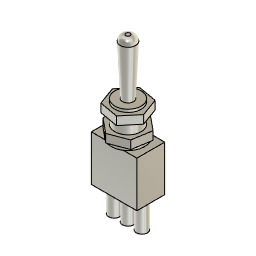
Zusammenbau V2 v20 (Autodesk Fusion 360 archive; units mm, degrees)
design "Schalter"
Autodesk Fusion 360 part; units mm, degrees
sketch "Skizze1" plane through (0, 0, 0) normal (0, 0, 1) x (1, 0, 0)
  line L0 (0, 0) -> (8.2, 0)
  line L1 (8.2, 0) -> (8.2, 5)
  line L2 (8.2, 5) -> (0, 5)
  line L3 (0, 5) -> (0, 0)
  dimension "d1" = 8.2
  dimension "d2" = 5
  constraint horizontal L0
  constraint vertical L1
  constraint horizontal L2
  constraint vertical L3
  constraint coincident L0.start L3.end
  measures "d1" distance of L0.start L0.end
  measures "d2" distance of L0.start L2.end
extrude "Extrusion1" add sketch "Skizze1" along normal blind 8.2
sketch "Skizze2" plane through (0, 0, 8.2) normal (0, 0, 1) x (-1, 0, 0)
  line L0 (0, -5) -> (0, 0)
  line L1 (0, 0) -> (-8.2, 0)
  line L2 (-8.2, 0) -> (-8.2, -5)
  line L3 (-8.2, -5) -> (0, -5)
  circle A0 centre (-4.1, -2.5) radius 3
  dimension "d5" = 6
  dimension "d6" = 2.5
  dimension "d38" = 4.1
  measures "d5" diameter of A0
  measures "d6" distance of L1 A0.centre
  measures "d38" distance of L0 A0.centre
extrude "Extrusion2" add sketch "Skizze2" along normal blind 0.5 contours L3 A0 | L1 L3 A0 | L1 A0
sketch "Skizze3" plane through (0, 0, 8.7) normal (0, 0, 1) x (-1, 0, 0)
  circle A0 centre (-4.1, -2.5) radius 3
  circle A1 centre (-4.1, -2.5) radius 2.375
  dimension "d9" = 4.75
  constraint concentric A0 A1
  measures "d9" diameter of A1
extrude "Extrusion3" add sketch "Skizze3" along normal blind 5.5 contours A1
sketch "Skizze4" plane through (0, 0, 14.2) normal (0, 0, 1) x (-1, 0, 0)
  circle A0 centre (-4.1, -2.5) radius 2.375
  circle A1 centre (-4.1, -2.5) radius 1.25
  dimension "d12" = 2.5
  constraint concentric A0 A1
  measures "d12" diameter of A1
sketch "Skizze5" plane through (0, 0, 0) normal (0, 0, -1) x (1, 0, 0)
  line L0 (0, 0) -> (0, -5)
  line L1 (0, -5) -> (8.2, -5)
  line L2 (8.2, -5) -> (8.2, 0)
  line L3 (8.2, 0) -> (0, 0)
  circle A0 centre (4.1, -2.5) radius 1
  circle A1 centre (6.6, -2.5) radius 1
  circle A2 centre (1.6, -2.5) radius 1
  dimension "d17" = 2
  dimension "d18" = 2.5
  dimension "d21" = 2.5
  dimension "d22" = 0
  dimension "d25" = -2.5
  dimension "d26" = 0
  dimension "d39" = 4.1
  measures "d17" diameter of A0
  measures "d18" distance of L1 A0.centre
  measures "d39" distance of L0 A0.centre
extrude "Extrusion5" add sketch "Skizze5" along normal blind 5 contours A0 | A1 | A2
sketch "Skizze6" plane through (0, 0, 8.7) normal (0, 0, 1) x (-1, 0, 0)
  circle A0 centre (-4.1, -2.5) radius 2.375
  circle A1 centre (-4.1, -2.5) radius 3
  line L0 (-7.3757, -3.7328) -> (-4.6702, -5.9532)
  line L1 (-4.6702, -5.9532) -> (-1.3945, -4.7204)
  line L2 (-1.3945, -4.7204) -> (-0.8243, -1.2672)
  line L3 (-0.8243, -1.2672) -> (-3.5298, 0.9532)
  line L4 (-3.5298, 0.9532) -> (-6.8055, -0.2796)
  line L5 (-6.8055, -0.2796) -> (-7.3757, -3.7328)
  point P0 (-4.1, -2.5)
  dimension "d29" = 3.5
  constraint coincident P0 A0.centre
  measures "d29" distance of L0.start P0
extrude "Extrusion6" add sketch "Skizze6" along normal blind 1.5 contours A1 | L0 L1 L2 L3 L4 L5
ref_plane "Arbeitsebene1" through (4.1, 2.5, 12.2) normal (0, 0, 1) x (-1, 0, 0)
sketch "Skizze8" plane through (4.1, 2.5, 12.2) normal (0, 0, 1) x (1, 0, 0)
  line L0 (-1.1793, 3.2572) -> (-3.4105, 0.6073)
  line L1 (-3.4105, 0.6073) -> (-2.2311, -2.6499)
  line L2 (-2.2311, -2.6499) -> (1.1793, -3.2572)
  line L3 (1.1793, -3.2572) -> (3.4105, -0.6073)
  line L4 (3.4105, -0.6073) -> (2.2311, 2.6499)
  line L5 (2.2311, 2.6499) -> (-1.1793, 3.2572)
  dimension "d40" = 3
  measures "d40" distance of origin L5
extrude "Extrusion9" add sketch "Skizze8" along normal blind 1.5
sketch "Skizze9" plane through (0, 0, 14.2) normal (0, 0, 1) x (-1, 0, 0)
  circle A0 centre (-4.1, -2.5) radius 2.375
  circle A1 centre (-4.1, -2.5) radius 1
  dimension "d43" = 2
  constraint concentric A0 A1
  measures "d43" diameter of A1
extrude "Extrusion10" add sketch "Skizze9" along normal blind 10 draft 2.5 contours A1
fillet "Abrundung2" radius 1 1 edges at (5.4394, 1.9805, 24.2)

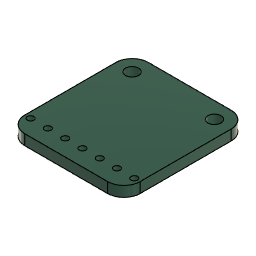
design "BME280"
Autodesk Fusion 360 part; units mm, degrees
sketch "Skizze1" plane through (0, 0, 0) normal (0, 0, 1) x (1, 0, 0)
  line L0 (2.5, 0) -> (15.28, 0)
  line L1 (17.78, 2.5) -> (17.78, 16.55)
  line L2 (15.28, 19.05) -> (2.5, 19.05)
  line L3 (0, 16.55) -> (0, 2.5)
  arc A0 (2.5, 19.05) -> (0, 16.55) centre (2.5, 16.55) ccw
  arc A1 (17.78, 16.55) -> (15.28, 19.05) centre (15.28, 16.55) ccw
  arc A2 (15.28, 0) -> (17.78, 2.5) centre (15.28, 2.5) ccw
  arc A3 (0, 2.5) -> (2.5, 0) centre (2.5, 2.5) ccw
  circle A4 centre (2.5, 16.55) radius 1
  circle A5 centre (15.2, 16.55) radius 1
  circle A6 centre (0.89, 2.5) radius 0.5
  circle A7 centre (3.5567, 2.5) radius 0.5
  circle A8 centre (6.2233, 2.5) radius 0.5
  circle A9 centre (8.89, 2.5) radius 0.5
  circle A10 centre (11.5567, 2.5) radius 0.5
  circle A11 centre (14.2233, 2.5) radius 0.5
  circle A12 centre (16.89, 2.5) radius 0.5
  point P0 (17.78, 0)
  dimension "d3" = 17.78
  dimension "d4" = 19.05
  dimension "d5" = 2.5
  dimension "d6" = 2
  dimension "d9" = 12.7
  dimension "d10" = 0
  dimension "d11" = 1
  dimension "d12" = 2.5
  dimension "d15" = 16
  dimension "d16" = 0
  dimension "d17" = 8.89
  constraint horizontal L0
  constraint vertical L1
  constraint horizontal L2
  constraint vertical L3
  constraint tangent L2 A0
  constraint tangent L3 A0
  constraint tangent L1 A1
  constraint tangent L2 A1
  constraint equal A0 A1
  constraint coincident P0 L0
  constraint coincident P0 L1
  constraint tangent L0 A2
  constraint tangent L1 A2
  constraint equal A0 A2
  constraint coincident origin L0
  constraint coincident origin L3
  constraint tangent L0 A3
  constraint tangent L3 A3
  constraint equal A0 A3
  constraint concentric A0 A4
  measures "d3" distance of origin P0
  measures "d4" distance of L0 L2
  measures "d5" radius of A0
  measures "d6" diameter of A4
  measures "d11" diameter of A6
  measures "d12" distance of L0 A6.centre
  measures "d17" distance of L3 A9.centre
extrude "Extrusion1" add sketch "Skizze1" along normal blind 1.6

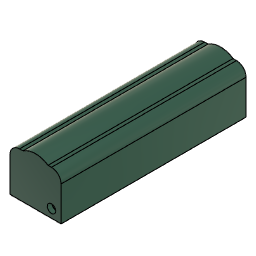
design "18650 Li-Ion Akku"
Autodesk Fusion 360 part; units mm, degrees
sketch "Skizze1" plane through (0, 0, 0) normal (0, 0, 1) x (1, 0, 0)
  line L0 (0, 0) -> (21.3, 0)
  line L1 (21.3, 0) -> (21.3, 77)
  line L2 (21.3, 77) -> (0, 77)
  line L3 (0, 77) -> (0, 0)
  dimension "d1" = 21.3
  dimension "d2" = 77
  constraint horizontal L0
  constraint vertical L1
  constraint horizontal L2
  constraint vertical L3
  constraint coincident L0.start L3.end
  measures "d1" distance of L0.start L0.end
  measures "d2" distance of L0.start L2.end
extrude "Extrusion1" add sketch "Skizze1" along normal blind 18.4
fillet "Abrundung1" radius 4 2 edges at (21.3, 38.5, 18.4) (0, 38.5, 18.4)
sketch "Skizze3" plane through (0, 0, 0) normal (0, -1, 0) x (1, 0, 0)
  arc A0 (4, 18.4) -> (0, 14.4) centre (4, 14.4) ccw
  line L0 (0, 14.4) -> (0, 0)
  line L1 (0, 0) -> (21.3, 0)
  line L2 (21.3, 0) -> (21.3, 14.4)
  arc A1 (21.3, 14.4) -> (17.3, 18.4) centre (17.3, 14.4) ccw
  line L3 (17.3, 18.4) -> (4, 18.4)
  circle A2 centre (10.65, 10.75) radius 9.25
  dimension "d10" = 18.5
  dimension "d11" = 10.75
  dimension "d12" = 10.65
  measures "d10" diameter of A2
  measures "d11" distance of L1 A2.centre
  measures "d12" distance of L0 A2.centre
extrude "Extrusion3" add sketch "Skizze3" against normal blind 77 contours L3 A2 picked at (9.7432, 18.797)
sketch "Skizze4" plane through (0, 0, 0) normal (0, -1, 0) x (1, 0, 0)
  arc A0 (4, 18.4) -> (0, 14.4) centre (4, 14.4) ccw
  line L0 (0, 14.4) -> (0, 0)
  line L1 (0, 0) -> (21.3, 0)
  line L2 (21.3, 0) -> (21.3, 14.4)
  arc A1 (21.3, 14.4) -> (17.3, 18.4) centre (17.3, 14.4) ccw
  line L3 (17.3, 18.4) -> (15.85, 18.4)
  arc A2 (15.85, 18.4) -> (5.45, 18.4) centre (10.65, 10.75) ccw
  line L4 (5.45, 18.4) -> (4, 18.4)
  circle A3 centre (17.3, 3.5) radius 1.75
  dimension "d15" = 3.5
  dimension "d16" = 4
  dimension "d17" = 3.5
  measures "d15" diameter of A3
  measures "d16" distance of L2 A3.centre
  measures "d17" distance of L1 A3.centre
extrude "Extrusion4" cut sketch "Skizze4" against normal blind 2 contours A3
sketch "Skizze5" plane through (0, 77, 0) normal (0, 1, 0) x (-1, 0, 0)
  arc A0 (0, 14.4) -> (-4, 18.4) centre (-4, 14.4) ccw
  line L0 (-4, 18.4) -> (-5.45, 18.4)
  arc A1 (-5.45, 18.4) -> (-15.85, 18.4) centre (-10.65, 10.75) ccw
  line L1 (-15.85, 18.4) -> (-17.3, 18.4)
  arc A2 (-17.3, 18.4) -> (-21.3, 14.4) centre (-17.3, 14.4) ccw
  line L2 (-21.3, 14.4) -> (-21.3, 0)
  line L3 (-21.3, 0) -> (0, 0)
  line L4 (0, 0) -> (0, 14.4)
  circle A3 centre (-4, 3.5) radius 1.75
  dimension "d20" = 3.5
  dimension "d21" = 4
  dimension "d22" = 3.5
  measures "d20" diameter of A3
  measures "d21" distance of L4 A3.centre
  measures "d22" distance of L3 A3.centre
extrude "Extrusion5" cut sketch "Skizze5" against normal blind 2 contours A3

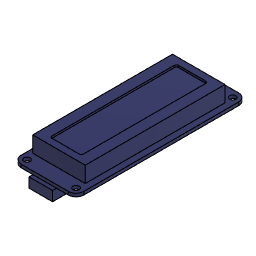
design "LCD1602 RGB Module"
Autodesk Fusion 360 part; units mm, degrees
sketch "Skizze1" plane through (0, 0, 0) normal (0, 0, 1) x (1, 0, 0)
  line L0 (4, 0) -> (28, 0)
  line L1 (32, 4) -> (32, 83)
  line L2 (28, 87) -> (4, 87)
  line L3 (0, 83) -> (0, 4)
  circle A0 centre (3.5, 3.5) radius 1.6
  circle A1 centre (28.5, 3.5) radius 1.6
  circle A2 centre (3.5, 83.5) radius 1.6
  circle A3 centre (28.5, 83.5) radius 1.6
  arc A4 (4, 87) -> (0, 83) centre (4, 83) ccw
  arc A5 (32, 83) -> (28, 87) centre (28, 83) ccw
  arc A6 (0, 4) -> (4, 0) centre (4, 4) ccw
  arc A7 (28, 0) -> (32, 4) centre (28, 4) ccw
  point P0 (32, 0)
  point P1 (0, 87)
  dimension "d1" = 32
  dimension "d2" = 87
  dimension "d3" = 3.2
  dimension "d4" = 3.5
  dimension "d5" = 3.5
  dimension "d8" = 25
  dimension "d9" = 80
  dimension "d10" = 4
  constraint horizontal L0
  constraint vertical L1
  constraint horizontal L2
  constraint vertical L3
  constraint coincident P1 L2
  constraint coincident P1 L3
  constraint tangent L2 A4
  constraint tangent L3 A4
  constraint tangent L1 A5
  constraint tangent L2 A5
  constraint equal A4 A5
  constraint coincident origin L0
  constraint coincident origin L3
  constraint tangent L0 A6
  constraint tangent L3 A6
  constraint equal A4 A6
  constraint coincident P0 L0
  constraint coincident P0 L1
  constraint tangent L0 A7
  constraint tangent L1 A7
  constraint equal A4 A7
  measures "d1" distance of origin P0
  measures "d2" distance of origin P1
  measures "d3" diameter of A0
  measures "d4" distance of L0 A0.centre
  measures "d5" distance of L3 A0.centre
  measures "d10" radius of A4
extrude "Extrusion1" add sketch "Skizze1" along normal blind 1.6
sketch "Skizze2" plane through (0, 0, 1.6) normal (0, 0, 1) x (-1, 0, 0)
  circle A0 centre (-28.5, -3.5) radius 1.6
  circle A1 centre (-3.5, -3.5) radius 1.6
  circle A2 centre (-3.5, -83.5) radius 1.6
  circle A3 centre (-28.5, -83.5) radius 1.6
  arc A4 (-28, 0) -> (-32, -4) centre (-28, -4) ccw
  line L0 (-32, -4) -> (-32, -83)
  arc A5 (-32, -83) -> (-28, -87) centre (-28, -83) ccw
  line L1 (-28, -87) -> (-4, -87)
  arc A6 (-4, -87) -> (0, -83) centre (-4, -83) ccw
  line L2 (0, -83) -> (0, -4)
  arc A7 (0, -4) -> (-4, 0) centre (-4, -4) ccw
  line L3 (-4, 0) -> (-28, 0)
  line L4 (-2.08, -7.8) -> (-28.88, -7.8)
  line L5 (-28.88, -7.8) -> (-28.88, -79.1)
  line L6 (-28.88, -79.1) -> (-2.08, -79.1)
  line L7 (-2.08, -79.1) -> (-2.08, -7.8)
  dimension "d13" = 26.8
  dimension "d14" = 71.3
  dimension "d15" = 7.8
  dimension "d16" = 2.08
  constraint horizontal L4
  constraint vertical L5
  constraint horizontal L6
  constraint vertical L7
  measures "d13" distance of L4.start L4.end
  measures "d14" distance of L4.start L6.end
  measures "d15" distance of L3 L4
  measures "d16" distance of L2 L7
extrude "Extrusion2" add sketch "Skizze2" along normal blind 8.1 contours L4 L5 L6 L7
sketch "Skizze3" plane through (0, 0, 9.7) normal (0, 0, 1) x (-1, 0, 0)
  line L0 (-2.08, -79.1) -> (-2.08, -7.8)
  line L1 (-2.08, -7.8) -> (-28.88, -7.8)
  line L2 (-28.88, -7.8) -> (-28.88, -79.1)
  line L3 (-28.88, -79.1) -> (-2.08, -79.1)
  line L4 (-8.48, -11.2) -> (-22.48, -11.2)
  line L5 (-23.48, -12.2) -> (-23.48, -74.7)
  line L6 (-22.48, -75.7) -> (-8.48, -75.7)
  line L7 (-7.48, -74.7) -> (-7.48, -12.2)
  arc A0 (-7.48, -12.2) -> (-8.48, -11.2) centre (-8.48, -12.2) ccw
  arc A1 (-22.48, -11.2) -> (-23.48, -12.2) centre (-22.48, -12.2) ccw
  arc A2 (-8.48, -75.7) -> (-7.48, -74.7) centre (-8.48, -74.7) ccw
  arc A3 (-23.48, -74.7) -> (-22.48, -75.7) centre (-22.48, -74.7) ccw
  point P0 (-7.48, -11.2)
  point P1 (-23.48, -11.2)
  point P2 (-7.48, -75.7)
  dimension "d19" = 16
  dimension "d20" = 64.5
  dimension "d21" = 3.4
  dimension "d22" = 5.4
  dimension "d23" = 1
  constraint horizontal L4
  constraint vertical L5
  constraint horizontal L6
  constraint vertical L7
  constraint coincident P0 L4
  constraint coincident P0 L7
  constraint tangent L4 A0
  constraint tangent L7 A0
  constraint coincident P1 L4
  constraint coincident P1 L5
  constraint tangent L4 A1
  constraint tangent L5 A1
  constraint equal A0 A1
  constraint coincident P2 L6
  constraint coincident P2 L7
  constraint tangent L6 A2
  constraint tangent L7 A2
  constraint equal A0 A2
  constraint tangent L5 A3
  constraint tangent L6 A3
  constraint equal A0 A3
  measures "d19" distance of P0 P1
  measures "d20" distance of P0 P2
  measures "d21" distance of L1 L4
  measures "d22" distance of L0 L7
  measures "d23" radius of A0
extrude "Extrusion3" cut sketch "Skizze3" against normal blind 1 contours L4 L5 L6 L7 A0 A1 A2 A3
sketch "Skizze4" plane through (0, 0, 1.6) normal (0, 0, 1) x (-1, 0, 0)
  line L0 (-2.08, -79.1) -> (-28.88, -79.1)
  line L1 (-28.88, -79.1) -> (-28.88, -7.8)
  line L2 (-28.88, -7.8) -> (-2.08, -7.8)
  line L3 (-2.08, -7.8) -> (-2.08, -79.1)
  circle A0 centre (-28.5, -3.5) radius 1.6
  circle A1 centre (-3.5, -3.5) radius 1.6
  circle A2 centre (-3.5, -83.5) radius 1.6
  circle A3 centre (-28.5, -83.5) radius 1.6
  arc A4 (-28, 0) -> (-32, -4) centre (-28, -4) ccw
  line L4 (-32, -4) -> (-32, -83)
  arc A5 (-32, -83) -> (-28, -87) centre (-28, -83) ccw
  line L5 (-28, -87) -> (-4, -87)
  arc A6 (-4, -87) -> (0, -83) centre (-4, -83) ccw
  line L6 (0, -83) -> (0, -4)
  arc A7 (0, -4) -> (-4, 0) centre (-4, -4) ccw
  line L7 (-4, 0) -> (-28, 0)
  line L8 (-7.48, -79.1) -> (-11.88, -83.5)
  line L9 (-11.88, -83.5) -> (-20.12, -83.5)
  line L10 (-20.12, -83.5) -> (-24.52, -79.1)
  dimension "d26" = 7.48
  dimension "d27" = 7.48
  dimension "d28" = 3.5
  dimension "d29" = 45
  dimension "d30" = 45
  constraint coincident L0 L8.start
  constraint parallel L0 L9
  constraint coincident L0 L10.end
  measures "d26" distance of L6 L8.start
  measures "d27" distance of L4 L10.end
  measures "d28" distance of L5 L9
  measures "d29" angle of L0 L8
  measures "d30" angle of L0 L10
extrude "Extrusion4" add sketch "Skizze4" along normal blind 3 contours L0 L8 L9 L10
sketch "Skizze5" plane through (0, 0, 0) normal (0, 0, -1) x (1, 0, 0)
  circle A0 centre (28.5, -3.5) radius 1.6
  circle A1 centre (3.5, -3.5) radius 1.6
  circle A2 centre (3.5, -83.5) radius 1.6
  circle A3 centre (28.5, -83.5) radius 1.6
  arc A4 (32, -4) -> (28, 0) centre (28, -4) ccw
  line L0 (28, 0) -> (4, 0)
  arc A5 (4, 0) -> (0, -4) centre (4, -4) ccw
  line L1 (0, -4) -> (0, -83)
  arc A6 (0, -83) -> (4, -87) centre (4, -83) ccw
  line L2 (4, -87) -> (28, -87)
  arc A7 (28, -87) -> (32, -83) centre (28, -83) ccw
  line L3 (32, -83) -> (32, -4)
  line L4 (2, -12) -> (5, -12)
  line L5 (5, -12) -> (5, -17)
  line L6 (5, -17) -> (2, -17)
  line L7 (2, -17) -> (2, -12)
  line L8 (30, -12) -> (30, -17)
  line L9 (30, -17) -> (27, -17)
  line L10 (27, -12) -> (30, -12)
  line L11 (27, -17) -> (27, -12)
  line L12 (5, -41) -> (5, -46)
  line L13 (5, -46) -> (2, -46)
  line L14 (2, -41) -> (5, -41)
  line L15 (2, -46) -> (2, -41)
  line L16 (30, -41) -> (30, -46)
  line L17 (30, -46) -> (27, -46)
  line L18 (27, -41) -> (30, -41)
  line L19 (27, -46) -> (27, -41)
  line L20 (5, -70) -> (5, -75)
  line L21 (5, -75) -> (2, -75)
  line L22 (2, -70) -> (5, -70)
  line L23 (2, -75) -> (2, -70)
  line L24 (30, -70) -> (30, -75)
  line L25 (30, -75) -> (27, -75)
  line L26 (27, -70) -> (30, -70)
  line L27 (27, -75) -> (27, -70)
  dimension "d33" = 3
  dimension "d34" = 5
  dimension "d35" = 12
  dimension "d36" = 2
  dimension "d39" = 25
  dimension "d40" = -58
  constraint horizontal L4
  constraint vertical L5
  constraint horizontal L6
  constraint vertical L7
  measures "d33" distance of L4.start L4.end
  measures "d34" distance of L4.start L6.end
  measures "d35" distance of L0 L4
  measures "d36" distance of L1 L7
extrude "Extrusion5" add sketch "Skizze5" along normal blind 2 contours L4 L5 L6 L7 | L8 L9 L10 L11 | L12 L13 L14 L15 | L16 L17 L18 L19 | L20 L21 L22 L23 | L24 L25 L26 L27
sketch "Skizze6" plane through (0, 0, 0) normal (0, 0, -1) x (1, 0, 0)
  line L0 (2, -17) -> (2, -12)
  line L1 (2, -12) -> (5, -12)
  line L2 (5, -12) -> (5, -17)
  line L3 (5, -17) -> (2, -17)
  line L4 (2, -75) -> (2, -70)
  line L5 (2, -70) -> (5, -70)
  line L6 (5, -70) -> (5, -75)
  line L7 (5, -75) -> (2, -75)
  line L8 (2, -46) -> (2, -41)
  line L9 (2, -41) -> (5, -41)
  line L10 (5, -41) -> (5, -46)
  line L11 (5, -46) -> (2, -46)
  line L12 (27, -17) -> (27, -12)
  line L13 (27, -12) -> (30, -12)
  line L14 (30, -12) -> (30, -17)
  line L15 (30, -17) -> (27, -17)
  line L16 (27, -75) -> (27, -70)
  line L17 (27, -70) -> (30, -70)
  line L18 (30, -70) -> (30, -75)
  line L19 (30, -75) -> (27, -75)
  line L20 (27, -46) -> (27, -41)
  line L21 (27, -41) -> (30, -41)
  line L22 (30, -41) -> (30, -46)
  line L23 (30, -46) -> (27, -46)
  circle A0 centre (28.5, -3.5) radius 1.6
  circle A1 centre (3.5, -3.5) radius 1.6
  circle A2 centre (3.5, -83.5) radius 1.6
  circle A3 centre (28.5, -83.5) radius 1.6
  arc A4 (32, -4) -> (28, 0) centre (28, -4) ccw
  line L24 (28, 0) -> (4, 0)
  arc A5 (4, 0) -> (0, -4) centre (4, -4) ccw
  line L25 (0, -4) -> (0, -83)
  arc A6 (0, -83) -> (4, -87) centre (4, -83) ccw
  line L26 (4, -87) -> (28, -87)
  arc A7 (28, -87) -> (32, -83) centre (28, -83) ccw
  line L27 (32, -83) -> (32, -4)
  line L28 (10, 2) -> (22, 2)
  line L29 (22, 2) -> (22, -8)
  line L30 (22, -8) -> (10, -8)
  line L31 (10, -8) -> (10, 2)
  dimension "d43" = 12
  dimension "d44" = 10
  dimension "d45" = 2
  dimension "d46" = 10
  constraint horizontal L28
  constraint vertical L29
  constraint horizontal L30
  constraint vertical L31
  measures "d43" distance of L28.start L28.end
  measures "d44" distance of L28.start L30.end
  measures "d45" distance of L24 L28
  measures "d46" distance of L25 L31
extrude "Extrusion6" add sketch "Skizze6" along normal blind 5 contours L24 L29 L30 L31 | L24 L28 L29 L31

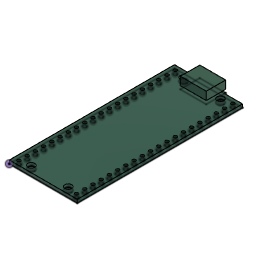
design "Pi Pico"
Autodesk Fusion 360 part; units mm, degrees
sketch "Skizze1" plane through (0, 0, 0) normal (0, 0, 1) x (1, 0, 0)
  line L0 (0, 0) -> (21, 0)
  line L1 (21, 0) -> (21, 51)
  line L2 (21, 51) -> (0, 51)
  line L3 (0, 51) -> (0, 0)
  circle A0 centre (4.8, 49) radius 1.05
  circle A1 centre (16.2, 49) radius 1.05
  circle A2 centre (4.8, 2) radius 1.05
  circle A3 centre (16.2, 2) radius 1.05
  line L4 (6.5, 52.3) -> (14.5, 52.3)
  line L5 (14.5, 52.3) -> (14.5, 46.3)
  line L6 (14.5, 46.3) -> (6.5, 46.3)
  line L7 (6.5, 46.3) -> (6.5, 52.3)
  circle A4 centre (1.61, 49.63) radius 0.5
  circle A5 centre (19.39, 49.63) radius 0.5
  circle A6 centre (1.61, 47.09) radius 0.5
  circle A7 centre (19.39, 47.09) radius 0.5
  circle A8 centre (1.61, 44.55) radius 0.5
  circle A9 centre (19.39, 44.55) radius 0.5
  circle A10 centre (1.61, 42.01) radius 0.5
  circle A11 centre (19.39, 42.01) radius 0.5
  circle A12 centre (1.61, 39.47) radius 0.5
  circle A13 centre (19.39, 39.47) radius 0.5
  circle A14 centre (1.61, 36.93) radius 0.5
  circle A15 centre (19.39, 36.93) radius 0.5
  circle A16 centre (1.61, 34.39) radius 0.5
  circle A17 centre (19.39, 34.39) radius 0.5
  circle A18 centre (1.61, 31.85) radius 0.5
  circle A19 centre (19.39, 31.85) radius 0.5
  circle A20 centre (1.61, 29.31) radius 0.5
  circle A21 centre (19.39, 29.31) radius 0.5
  circle A22 centre (1.61, 26.77) radius 0.5
  circle A23 centre (19.39, 26.77) radius 0.5
  circle A24 centre (1.61, 24.23) radius 0.5
  circle A25 centre (19.39, 24.23) radius 0.5
  circle A26 centre (1.61, 21.69) radius 0.5
  circle A27 centre (19.39, 21.69) radius 0.5
  circle A28 centre (1.61, 19.15) radius 0.5
  circle A29 centre (19.39, 19.15) radius 0.5
  circle A30 centre (1.61, 16.61) radius 0.5
  circle A31 centre (19.39, 16.61) radius 0.5
  circle A32 centre (1.61, 14.07) radius 0.5
  circle A33 centre (19.39, 14.07) radius 0.5
  circle A34 centre (1.61, 11.53) radius 0.5
  circle A35 centre (19.39, 11.53) radius 0.5
  circle A36 centre (1.61, 8.99) radius 0.5
  circle A37 centre (19.39, 8.99) radius 0.5
  circle A38 centre (1.61, 6.45) radius 0.5
  circle A39 centre (19.39, 6.45) radius 0.5
  circle A40 centre (1.61, 3.91) radius 0.5
  circle A41 centre (19.39, 3.91) radius 0.5
  circle A42 centre (1.61, 1.37) radius 0.5
  circle A43 centre (19.39, 1.37) radius 0.5
  dimension "d1" = 21
  dimension "d2" = 51
  dimension "d3" = 2.1
  dimension "d4" = 4.8
  dimension "d5" = 2
  dimension "d8" = 11.4
  dimension "d9" = -47
  dimension "d10" = 8
  dimension "d11" = 6
  dimension "d12" = 1.3
  dimension "d13" = 6.5
  dimension "d20" = 1
  dimension "d21" = 1.37
  dimension "d22" = 1.61
  dimension "d25" = 17.78
  dimension "d26" = -2.54
  constraint horizontal L0
  constraint vertical L1
  constraint horizontal L2
  constraint vertical L3
  constraint coincident L0.start L3.end
  constraint horizontal L4
  constraint vertical L5
  constraint horizontal L6
  constraint vertical L7
  measures "d1" distance of L0.start L0.end
  measures "d2" distance of L0.start L2.end
  measures "d3" diameter of A0
  measures "d4" distance of L3 A0.centre
  measures "d5" distance of L2 A0.centre
  measures "d10" distance of L4.start L4.end
  measures "d11" distance of L4.start L6.end
  measures "d12" distance of L2 L4
  measures "d13" distance of L1 L5
  measures "d20" diameter of A4
  measures "d21" distance of L2 A4.centre
  measures "d22" distance of L3 A4.centre
extrude "Extrusion4" add sketch "Skizze1" along normal blind 1 contours L0 L1 L2 L3 L5 L6 L7
extrude "Extrusion2" add sketch "Skizze1" along normal blind 3.5 contours L2 L4 L5 L7 | L2 L5 L6 L7
extrude "Extrusion3" cut sketch "Skizze1" along normal blind 1 contours L2 L4 L5 L7

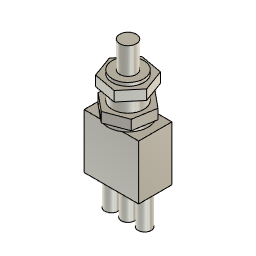
design "Taster"
Autodesk Fusion 360 part; units mm, degrees
sketch "Skizze1" plane through (0, 0, 0) normal (0, 0, 1) x (1, 0, 0)
  line L0 (0, 0) -> (8.2, 0)
  line L1 (8.2, 0) -> (8.2, 5)
  line L2 (8.2, 5) -> (0, 5)
  line L3 (0, 5) -> (0, 0)
  dimension "d1" = 8.2
  dimension "d2" = 5
  constraint horizontal L0
  constraint vertical L1
  constraint horizontal L2
  constraint vertical L3
  constraint coincident L0.start L3.end
  measures "d1" distance of L0.start L0.end
  measures "d2" distance of L0.start L2.end
extrude "Extrusion1" add sketch "Skizze1" along normal blind 8.2
sketch "Skizze2" plane through (0, 0, 8.2) normal (0, 0, 1) x (-1, 0, 0)
  line L0 (0, -5) -> (0, 0)
  line L1 (0, 0) -> (-8.2, 0)
  line L2 (-8.2, 0) -> (-8.2, -5)
  line L3 (-8.2, -5) -> (0, -5)
  circle A0 centre (-4.1, -2.5) radius 3
  dimension "d5" = 6
  dimension "d6" = 2.5
  dimension "d38" = 4.1
  measures "d5" diameter of A0
  measures "d6" distance of L1 A0.centre
  measures "d38" distance of L0 A0.centre
extrude "Extrusion2" add sketch "Skizze2" along normal blind 0.5 contours L3 A0 | L1 L3 A0 | L1 A0
sketch "Skizze3" plane through (0, 0, 8.7) normal (0, 0, 1) x (-1, 0, 0)
  circle A0 centre (-4.1, -2.5) radius 3
  circle A1 centre (-4.1, -2.5) radius 2.375
  dimension "d9" = 4.75
  constraint concentric A0 A1
  measures "d9" diameter of A1
extrude "Extrusion3" add sketch "Skizze3" along normal blind 5.5 contours A1
sketch "Skizze4" plane through (0, 0, 14.2) normal (0, 0, 1) x (-1, 0, 0)
  circle A0 centre (-4.1, -2.5) radius 2.375
  circle A1 centre (-4.1, -2.5) radius 1.25
  dimension "d12" = 2.5
  constraint concentric A0 A1
  measures "d12" diameter of A1
sketch "Skizze5" plane through (0, 0, 0) normal (0, 0, -1) x (1, 0, 0)
  line L0 (0, 0) -> (0, -5)
  line L1 (0, -5) -> (8.2, -5)
  line L2 (8.2, -5) -> (8.2, 0)
  line L3 (8.2, 0) -> (0, 0)
  circle A0 centre (4.1, -2.5) radius 1
  circle A1 centre (6.6, -2.5) radius 1
  circle A2 centre (1.6, -2.5) radius 1
  dimension "d17" = 2
  dimension "d18" = 2.5
  dimension "d21" = 2.5
  dimension "d22" = 0
  dimension "d25" = -2.5
  dimension "d26" = 0
  dimension "d39" = 4.1
  measures "d17" diameter of A0
  measures "d18" distance of L1 A0.centre
  measures "d39" distance of L0 A0.centre
extrude "Extrusion5" add sketch "Skizze5" along normal blind 5 contours A0 | A1 | A2
sketch "Skizze6" plane through (0, 0, 8.7) normal (0, 0, 1) x (-1, 0, 0)
  circle A0 centre (-4.1, -2.5) radius 2.375
  circle A1 centre (-4.1, -2.5) radius 3
  line L0 (-7.3757, -3.7328) -> (-4.6702, -5.9532)
  line L1 (-4.6702, -5.9532) -> (-1.3945, -4.7204)
  line L2 (-1.3945, -4.7204) -> (-0.8243, -1.2672)
  line L3 (-0.8243, -1.2672) -> (-3.5298, 0.9532)
  line L4 (-3.5298, 0.9532) -> (-6.8055, -0.2796)
  line L5 (-6.8055, -0.2796) -> (-7.3757, -3.7328)
  point P0 (-4.1, -2.5)
  dimension "d29" = 3.5
  constraint coincident P0 A0.centre
  measures "d29" distance of L0.start P0
extrude "Extrusion6" add sketch "Skizze6" along normal blind 1.5 contours A1 | L0 L1 L2 L3 L4 L5
extrude "Extrusion7" add sketch "Skizze4" along normal blind 4 contours A1
ref_plane "Arbeitsebene1" through (4.1, 2.5, 12.2) normal (0, 0, 1) x (-1, 0, 0)
sketch "Skizze8" plane through (4.1, 2.5, 12.2) normal (0, 0, 1) x (1, 0, 0)
  line L0 (-1.1793, 3.2572) -> (-3.4105, 0.6073)
  line L1 (-3.4105, 0.6073) -> (-2.2311, -2.6499)
  line L2 (-2.2311, -2.6499) -> (1.1793, -3.2572)
  line L3 (1.1793, -3.2572) -> (3.4105, -0.6073)
  line L4 (3.4105, -0.6073) -> (2.2311, 2.6499)
  line L5 (2.2311, 2.6499) -> (-1.1793, 3.2572)
  dimension "d40" = 3
  measures "d40" distance of origin L5
extrude "Extrusion9" add sketch "Skizze8" along normal blind 1.5

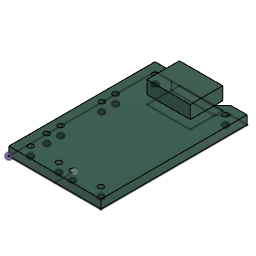
design "TP4056 Battery Charger"
Autodesk Fusion 360 part; units mm, degrees
sketch "Skizze1" plane through (0, 0, 0) normal (0, 0, 1) x (1, 0, 0)
  line L0 (0, 0) -> (17, 0)
  line L1 (17, 0) -> (17, 27)
  line L2 (17, 27) -> (0, 27)
  line L3 (0, 27) -> (0, 0)
  line L4 (14, 27) -> (12.5, 25.5)
  line L5 (12.5, 25.5) -> (4.5, 25.5)
  line L6 (4.5, 25.5) -> (3, 27)
  line L7 (4.5, 27) -> (12.5, 27)
  line L8 (12.5, 27) -> (12.5, 21)
  line L9 (12.5, 21) -> (4.5, 21)
  line L10 (4.5, 21) -> (4.5, 27)
  circle A0 centre (2, 25) radius 0.5
  circle A1 centre (15, 25) radius 0.5
  circle A2 centre (2, 2) radius 0.5
  circle A3 centre (15, 2) radius 0.5
  circle A4 centre (7.23, 2) radius 0.5
  circle A5 centre (9.77, 2) radius 0.5
  line L11 (8.5, 0) -> (8.5, 3.6203)
  circle A6 centre (1.5, 5.5) radius 0.5
  circle A7 centre (1.5, 8.04) radius 0.5
  circle A8 centre (1.5, 15.66) radius 0.5
  circle A9 centre (1.5, 18.2) radius 0.5
  dimension "d1" = 17
  dimension "d2" = 27
  dimension "d3" = 3
  dimension "d4" = 3
  dimension "d5" = 45
  dimension "d6" = 45
  dimension "d7" = 1.5
  dimension "d8" = 8
  dimension "d9" = 6
  dimension "d10" = 4.5
  dimension "d17" = 1
  dimension "d18" = 2
  dimension "d19" = 2
  dimension "d22" = 13
  dimension "d23" = -23
  dimension "d24" = 1
  dimension "d25" = 2
  dimension "d28" = 2.54
  dimension "d29" = 0
  dimension "d30" = 1
  dimension "d31" = 5.5
  dimension "d32" = 1.5
  dimension "d35" = 0
  dimension "d36" = 2.54
  dimension "d39" = 0
  dimension "d40" = 10.16
  constraint horizontal L0
  constraint vertical L1
  constraint horizontal L2
  constraint vertical L3
  constraint coincident L0.start L3.end
  constraint coincident L2 L4.start
  constraint perpendicular L1 L5
  constraint coincident L2 L6.end
  constraint horizontal L7
  constraint vertical L8
  constraint horizontal L9
  constraint vertical L10
  constraint collinear L2 L7
  constraint midpoint L0 L11.start
  constraint perpendicular L0 L11
  constraint symmetric A4 A5 L11
  measures "d1" distance of L0.start L0.end
  measures "d2" distance of L0.start L2.end
  measures "d3" distance of L2.end L6.end
  measures "d4" distance of L1.end L4.start
  measures "d5" angle of L2 L4
  measures "d6" angle of L2 L6
  measures "d7" distance of L2 L5
  measures "d8" distance of L7.start L7.end
  measures "d9" distance of L7.start L9.end
  measures "d10" distance of L3 L10
  measures "d17" diameter of A0
  measures "d18" distance of L3 A0.centre
  measures "d19" distance of L2 A0.centre
  measures "d24" diameter of A4
  measures "d25" distance of L0 A4.centre
  measures "d30" diameter of A6
  measures "d31" distance of L0 A6.centre
  measures "d32" distance of L3 A6.centre
extrude "Extrusion2" add sketch "Skizze1" along normal blind 4 contours L2 L5 L7 L8 L10 | L5 L8 L9 L10
extrude "Extrusion3" cut sketch "Skizze1" along normal blind 1.6 contours L2 L5 L7 L8 L10
extrude "Extrusion4" add sketch "Skizze1" along normal blind 1.6 contours L0 L1 L2 L3 L4 L6 L8 L9 L10
sketch "Skizze2" plane through (0, 0, 1.6) normal (0, 0, 1) x (-1, 0, 0)
  circle A0 centre (-1.5, -15.66) radius 0.5
  circle A1 centre (-2, -2) radius 0.5
  circle A2 centre (-1.5, -8.04) radius 0.5
  circle A3 centre (-15, -25) radius 0.5
  circle A4 centre (-1.5, -18.2) radius 0.5
  circle A5 centre (-7.23, -2) radius 0.5
  circle A6 centre (-1.5, -5.5) radius 0.5
  circle A7 centre (-15, -2) radius 0.5
  circle A8 centre (-9.77, -2) radius 0.5
  circle A9 centre (-2, -25) radius 0.5
  line L0 (-4.5, -21) -> (-4.5, -25.5)
  line L1 (-4.5, -25.5) -> (-3, -27)
  line L2 (-3, -27) -> (0, -27)
  line L3 (0, -27) -> (0, 0)
  line L4 (0, 0) -> (-17, 0)
  line L5 (-17, 0) -> (-17, -27)
  line L6 (-17, -27) -> (-14, -27)
  line L7 (-14, -27) -> (-12.5, -25.5)
  line L8 (-12.5, -25.5) -> (-12.5, -21)
  line L9 (-12.5, -21) -> (-4.5, -21)
  line L10 (-4.75, -3.5) -> (-12.25, -3.5)
  line L11 (-12.25, -3.5) -> (-12.25, 7.5)
  line L12 (-12.25, 7.5) -> (-4.75, 7.5)
  line L13 (-4.75, 7.5) -> (-4.75, -3.5)
  line L14 (-4.75, 0) -> (-12.25, 0)
  line L15 (0, 0) -> (-17, 0)
  dimension "d43" = 7.5
  dimension "d44" = 11
  dimension "d45" = 3.5
  constraint horizontal L10
  constraint vertical L11
  constraint horizontal L12
  constraint vertical L13
  constraint coincident L13 L14.start
  constraint coincident L11 L14.end
  constraint perpendicular L11 L14
  constraint midpoint L14 L15
  measures "d43" distance of L10.start L10.end
  measures "d44" distance of L10.start L12.end
  measures "d45" distance of L10 L14
extrude "Extrusion5" [rolled back] along distance 6 taper angle 0

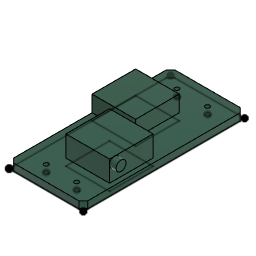
design "MT3608 Step-up"
Autodesk Fusion 360 part; units mm, degrees
sketch "Skizze1" plane through (0, 0, 0) normal (0, 0, 1) x (1, 0, 0)
  line L0 (1, 0) -> (16, 0)
  line L1 (17, 1) -> (17, 36)
  line L2 (16, 37) -> (1, 37)
  line L3 (0, 36) -> (0, 1)
  circle A0 centre (5, 33.5) radius 0.5
  circle A1 centre (12, 33.5) radius 0.5
  circle A2 centre (5, 3.5) radius 0.5
  circle A3 centre (12, 3.5) radius 0.5
  line L4 (0, 29) -> (10, 29)
  line L5 (10, 29) -> (10, 19)
  line L6 (10, 19) -> (0, 19)
  line L7 (0, 19) -> (0, 29)
  line L8 (16, 7) -> (6, 7)
  line L9 (6, 7) -> (6, 17)
  line L10 (6, 17) -> (16, 17)
  line L11 (16, 17) -> (16, 7)
  line L12 (1, 37) -> (0, 36)
  line L13 (17, 36) -> (16, 37)
  line L14 (1, 0) -> (0, 1)
  line L15 (16, 0) -> (17, 1)
  point P0 (17, 0)
  point P1 (17, 37)
  point P2 (0, 37)
  dimension "d1" = 17
  dimension "d2" = 37
  dimension "d3" = 1
  dimension "d4" = 5
  dimension "d5" = 3.5
  dimension "d8" = 7
  dimension "d9" = -30
  dimension "d10" = 10
  dimension "d11" = 10
  dimension "d12" = 8
  dimension "d13" = 10
  dimension "d14" = 10
  dimension "d15" = 7
  dimension "d16" = 1
  dimension "d28" = 1
  dimension "d29" = 1
  dimension "d30" = 1
  dimension "d31" = 1
  dimension "d32" = 1
  dimension "d33" = 1
  dimension "d34" = 1
  dimension "d35" = 1
  constraint horizontal L0
  constraint vertical L1
  constraint horizontal L2
  constraint vertical L3
  constraint horizontal L4
  constraint vertical L5
  constraint horizontal L6
  constraint vertical L7
  constraint coincident L3 L4.start
  constraint horizontal L8
  constraint vertical L9
  constraint horizontal L10
  constraint vertical L11
  constraint coincident P2 L2
  constraint coincident P2 L3
  constraint coincident P1 L1
  constraint coincident P1 L2
  constraint coincident origin L0
  constraint coincident origin L3
  constraint coincident P0 L0
  constraint coincident P0 L1
  measures "d1" distance of origin P0
  measures "d2" distance of origin P2
  measures "d3" diameter of A0
  measures "d4" distance of L3 A0.centre
  measures "d5" distance of L2 A0.centre
  measures "d10" distance of L4.start L4.end
  measures "d11" distance of L4.start L6.end
  measures "d12" distance of L2 L4
  measures "d13" distance of L8.start L8.end
  measures "d14" distance of L8.start L10.end
  measures "d15" distance of L0 L8
  measures "d16" distance of L1 L11
  measures "d28" distance of P2 L2.end
  measures "d29" distance of P2 L3.start
  measures "d30" distance of P1 L1.end
  measures "d31" distance of P1 L2.start
  measures "d32" distance of origin L0.start
  measures "d33" distance of origin L3.end
  measures "d34" distance of P0 L0.end
  measures "d35" distance of P0 L1.start
extrude "Extrusion1" add sketch "Skizze1" along normal blind 1.6 contours L0 L1 L2 L3 L4 L5 L6 L12 L13 L14 L15
extrude "Extrusion2" add sketch "Skizze1" along normal blind 5.3 contours L3 L4 L5 L6 L7
extrude "Extrusion3" add sketch "Skizze1" along normal blind 6.4 contours L8 L9 L10 L11
sketch "Skizze2" plane through (16, 0, 0) normal (1, 0, 0) x (0, 1, 0)
  line L0 (17, 1.6) -> (17, 6.4)
  line L1 (17, 6.4) -> (7, 6.4)
  line L2 (7, 6.4) -> (7, 1.6)
  circle A0 centre (8.15, 5.25) radius 1.15
  line L3 (7, 1.6) -> (17, 1.6)
  dimension "d23" = 2.3
  dimension "d24" = 1.15
  dimension "d25" = 1.15
  measures "d23" diameter of A0
  measures "d24" distance of L2 A0.centre
  measures "d25" distance of L1 A0.centre
extrude "Extrusion4" add sketch "Skizze2" along normal blind 1.5 contours A0
equation "d29 = d28"
equation "d31 = d30"
equation "d33 = d32"
equation "d35 = d34"
